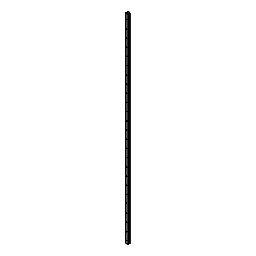
Linear guide rail v1 (Autodesk Fusion 360 design; units mm, degrees)
Autodesk Fusion 360 part; units mm, degrees
sketch "Sketch1" plane through (0, 0, 0) normal (0, 0, 1) x (1, 0, 0)
  line L0 (10, -8.75) -> (-10, -8.75)
  line L1 (10, -8.75) -> (10, -4.15)
  line L2 (0, 0) -> (12.5, 0) construction
  line L3 (10, -4.15) -> (5.85, 0)
  line L4 (5.85, 0) -> (5.85, 2)
  line L5 (9.9, -8.75) -> (10, -8.65)
  line L6 (9.9, -8.75) -> (10.0414, -8.75) construction
  line L7 (10, 6.45) -> (10, 4.95)
  line L8 (10, 6.45) -> (6.5, 8.75)
  line L9 (10, 4.95) -> (5.85, 2)
  line L10 (-10, -8.75) -> (10, -8.75) construction
  line L11 (-9.9, -8.75) -> (-10, -8.65)
  line L12 (-10, -8.75) -> (-10, -4.15)
  line L13 (-10, -4.15) -> (-5.85, 0)
  line L14 (-5.85, 0) -> (-5.85, 2)
  line L15 (-10, 4.95) -> (-5.85, 2)
  line L16 (-10, 6.45) -> (-6.5, 8.75)
  line L17 (-10, 6.45) -> (-10, 4.95)
  line L18 (-6.5, 8.75) -> (6.5, 8.75)
  dimension "d8" = 20
  dimension "d9" = 4.6
  dimension "d16" = 45
  dimension "d18" = 1.5
  dimension "d19" = 2
  dimension "d20" = 2
  dimension "d21" = 1.5
  dimension "d22" = 4.6
  dimension "d23" = 13
  constraint perpendicular L0 L1
  constraint coincident L2.start origin
  constraint coincident L2 L3.end
  constraint perpendicular L2 L4
  constraint coincident L0 L5.start
  constraint horizontal L6
  constraint coincident L1 L5.end
  constraint horizontal L18
  measures "d8" distance of L0.start L0.end
  measures "d9" distance of L0.start L1.end
  measures "d16" angle of L5 L6
  measures "d18" distance of L7.start L7.end
  measures "d19" distance of L3.end L4.end
  measures "d20" distance of L13.end L14.end
  measures "d21" distance of L15.start L16.start
  measures "d22" distance of L0.end L12.end
  measures "d23" distance of L8.end L16.end
extrude "Extrude1" add sketch "Sketch1" along normal blind 1500 contours L0 L1 L3 L4 L5 L7 L8 L9 L11 L12 L13 L14 L15 L16 L17 L18
sketch "Sketch2" plane through (0, 8.75, 0) normal (0, 1, 0) x (-1, 0, 0)
  line L0 (-6.5, 0) -> (6.5, 0)
  line L1 (6.5, 0) -> (6.5, 1500)
  line L2 (6.5, 1500) -> (-6.5, 1500)
  line L3 (-6.5, 1500) -> (-6.5, 0)
  line L4 (0, 0) -> (0, 20) construction
  circle A0 centre (0, 20) radius 4.75
  circle A1 centre (0, 20) radius 3
  dimension "d26" = 20
  dimension "d27" = 9.5
  dimension "d28" = 6
  constraint coincident L4.start origin
  constraint perpendicular L0 L4
  constraint coincident L4.end A0.centre
  constraint concentric A0 A1
  measures "d26" distance of L4.start L4.end
  measures "d27" diameter of A0
  measures "d28" diameter of A1
extrude "Extrude2" cut sketch "Sketch2" against normal blind 8.5 contours A0 | A1
extrude "Extrude3" cut sketch "Sketch2" against normal blind 17.5 contours A1
pattern_linear "R-Pattern1" count 25 spacing 60 along (0, 0, 1) of "Extrude2", "Extrude3"
